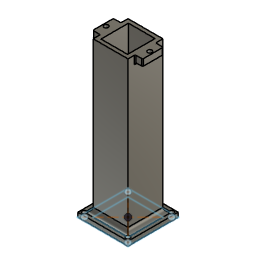
AUT Booster Seat v2 (Autodesk Fusion 360 design; units mm, degrees)
Autodesk Fusion 360 part; units mm, degrees
sketch "Sketch1" plane through (0, 0, 0) normal (0, 0, 1) x (1, 0, 0)
  circle A0 centre (-25.4, 25.4) radius 2.55
  circle A1 centre (25.4, 25.4) radius 2.55
  circle A2 centre (-25.4, -25.4) radius 2.55
  circle A3 centre (25.4, -25.4) radius 2.55
  line L0 (29.21, 29.21) -> (-29.21, 29.21)
  line L1 (-29.21, 29.21) -> (-29.21, -29.21)
  line L2 (-29.21, -29.21) -> (29.21, -29.21)
  line L3 (29.21, -29.21) -> (29.21, 29.21)
  line L4 (29.21, 29.21) -> (-29.21, -29.21) construction
  line L5 (-29.21, 29.21) -> (29.21, -29.21) construction
  line L6 (20.32, 20.32) -> (-20.32, 20.32)
  line L7 (-20.32, 20.32) -> (-20.32, -20.32)
  line L8 (-20.32, -20.32) -> (20.32, -20.32)
  line L9 (20.32, -20.32) -> (20.32, 20.32)
  line L10 (20.32, 20.32) -> (-20.32, -20.32) construction
  line L11 (-20.32, 20.32) -> (20.32, -20.32) construction
  dimension "d1" = 5.1
  dimension "d2" = 5.1
  dimension "d3" = 5.1
  dimension "d4" = 5.1
  constraint horizontal L0
  constraint perpendicular L0 L1
  constraint parallel L0 L2
  constraint parallel L1 L3
  constraint coincident L4 origin
  constraint coincident L5 origin
  constraint horizontal L6
  constraint perpendicular L6 L7
  constraint parallel L6 L8
  constraint parallel L7 L9
  constraint coincident L10 origin
  constraint coincident L11 origin
  constraint coincident L4 L6.start
  measures "d1" diameter of A0
  measures "d2" diameter of A1
  measures "d3" diameter of A2
  measures "d4" diameter of A3
extrude "Extrude1" add sketch "Sketch1" along normal blind 5 contours L0 L1 L2 L3 | L6 L7 L8 L9
sketch "Sketch2" plane through (0, 0, 5) normal (0, 0, 1) x (-1, 0, 0)
  circle A0 centre (-25.4, -25.4) radius 2.55
  circle A1 centre (25.4, 25.4) radius 2.55
  circle A2 centre (-25.4, 25.4) radius 2.55
  circle A3 centre (25.4, -25.4) radius 2.55
  line L0 (-29.21, 29.21) -> (-29.21, -29.21)
  line L1 (-29.21, -29.21) -> (29.21, -29.21)
  line L2 (29.21, -29.21) -> (29.21, 29.21)
  line L3 (29.21, 29.21) -> (-29.21, 29.21)
  line L4 (20.3, 20.3) -> (-20.3, 20.3)
  line L5 (-20.3, 20.3) -> (-20.3, -20.3)
  line L6 (-20.3, -20.3) -> (20.3, -20.3)
  line L7 (20.3, -20.3) -> (20.3, 20.3)
  line L8 (20.3, 20.3) -> (-20.3, -20.3) construction
  line L9 (-20.3, 20.3) -> (20.3, -20.3) construction
  constraint horizontal L4
  constraint perpendicular L4 L5
  constraint parallel L4 L6
  constraint parallel L5 L7
  constraint coincident L8 origin
  constraint coincident L9 origin
extrude "Extrude2" add sketch "Sketch2" along normal blind 175 contours L4 L5 L6 L7
fillet "Fillet1" radius 5 4 edges at (20.3, 0, 5) (0, -20.3, 5) (0, 20.3, 5) (-20.3, 0, 5)
sketch "Sketch3" plane through (0, 0, 180) normal (0, 0, 1) x (-1, 0, 0)
  line L0 (20.3, -20.3) -> (20.3, 20.3)
  line L1 (20.3, 20.3) -> (-20.3, 20.3)
  line L2 (-20.3, 20.3) -> (-20.3, -20.3)
  line L3 (-20.3, -20.3) -> (20.3, -20.3)
  line L4 (29, 12) -> (-29, 12)
  line L5 (-29, 12) -> (-29, -12)
  line L6 (-29, -12) -> (29, -12)
  line L7 (29, -12) -> (29, 12)
  line L8 (29, 12) -> (-29, -12) construction
  line L9 (-29, 12) -> (29, -12) construction
  circle A0 centre (-25.4, 0) radius 2.55
  circle A1 centre (25.4, 0) radius 2.55
  dimension "d11" = 5.1
  dimension "d12" = 5.1
  constraint horizontal L4
  constraint perpendicular L4 L5
  constraint parallel L4 L6
  constraint parallel L5 L7
  constraint coincident L8 origin
  constraint coincident L9 origin
  measures "d11" diameter of A0
  measures "d12" diameter of A1
extrude "Extrude3" add sketch "Sketch3" against normal blind 5 contours L0 L4 L6 L7 | L2 L4 L5 L6
fillet "Fillet2" radius 1 8 edges at (-20.3, -12, 177.5) (-29, -12, 177.5) (-29, 12, 177.5) (-20.3, 12, 177.5) (29, -12, 177.5) (20.3, -12, 177.5) (29, 12, 177.5) (20.3, 12, 177.5)
move_face "MoveFace1" by (0, 0, -2.54) 2 faces at (-24.8365, 8.8476, 175) (24.8365, 8.8476, 175)
fillet "Fillet3" radius 2 2 edges at (-20.3, 0, 172.46) (20.3, 0, 172.46)
sketch "Sketch4" plane through (0, 0, 180) normal (0, 0, 1) x (-1, 0, 0)
  circle A0 centre (25.4, 0) radius 2.55
  circle A1 centre (-25.4, 0) radius 2.55
  arc A2 (-29, -11) -> (-28, -12) centre (-28, -11) ccw
  line L0 (-28, -12) -> (-21.3, -12)
  arc A3 (-20.3, -13) -> (-21.3, -12) centre (-21.3, -13) ccw
  line L1 (-20.3, -13) -> (-20.3, -20.3)
  line L2 (-20.3, -20.3) -> (20.3, -20.3)
  line L3 (20.3, -20.3) -> (20.3, -13)
  arc A4 (21.3, -12) -> (20.3, -13) centre (21.3, -13) ccw
  line L4 (21.3, -12) -> (28, -12)
  arc A5 (28, -12) -> (29, -11) centre (28, -11) ccw
  line L5 (29, -11) -> (29, 11)
  arc A6 (29, 11) -> (28, 12) centre (28, 11) ccw
  line L6 (28, 12) -> (21.3, 12)
  arc A7 (20.3, 13) -> (21.3, 12) centre (21.3, 13) ccw
  line L7 (20.3, 13) -> (20.3, 20.3)
  line L8 (20.3, 20.3) -> (-20.3, 20.3)
  line L9 (-20.3, 20.3) -> (-20.3, 13)
  arc A8 (-21.3, 12) -> (-20.3, 13) centre (-21.3, 13) ccw
  line L10 (-21.3, 12) -> (-28, 12)
  arc A9 (-28, 12) -> (-29, 11) centre (-28, 11) ccw
  line L11 (-29, 11) -> (-29, -11)
  line L12 (-15.4745, -15.9919) -> (15.4745, -15.9919)
  line L13 (15.4745, -15.9919) -> (15.4745, 15.9919)
  line L14 (15.4745, 15.9919) -> (-15.4745, 15.9919)
  line L15 (-15.4745, 15.9919) -> (-15.4745, -15.9919)
  line L16 (-15.4745, -15.9919) -> (15.4745, 15.9919) construction
  line L17 (15.4745, -15.9919) -> (-15.4745, 15.9919) construction
  constraint horizontal L12
  constraint perpendicular L12 L13
  constraint parallel L12 L14
  constraint parallel L13 L15
  constraint coincident L16 origin
  constraint coincident L17 origin
extrude "Extrude4" cut sketch "Sketch4" against normal blind 198.12 contours L12 L13 L14 L15
